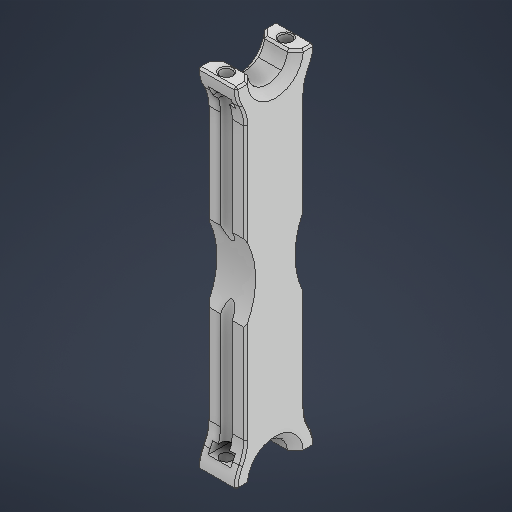
# Autodesk Inventor part: gaffel
Saved by Autodesk Inventor 2026.3 (Build 303398000, 398)
## iProperties
Created: 2026-05-02
Part Number: gaffel
Material: Generic
Document SubType Name: Modeling
Designer: frede
Density: 1 g/cm^3
Appearance: Default
Author: frede
Autodesk Inventor part; units mm, degrees
ref_plane "YZ Plane" through (0, 0, 0) normal (1, 0, 0) x (0, 1, 0)
sketch "Sketch1" plane through (0, 0, 0) normal (1, 0, 0) x (0, 1, 0)
  circle A0 centre (0, 0) radius 5.1
  circle A1 centre (88.4, 0) radius 5.1
  arc A2 (6.6144, 7.5) -> (6.6144, -7.5) centre (0, 0) ccw
  arc A3 (81.7856, -7.5) -> (81.7856, 7.5) centre (88.4, 0) ccw
  line L0 (10, 0) -> (78.4, 0)
  line L1 (81.7856, -7.5) -> (6.6144, -7.5)
  line L2 (6.6144, 7.5) -> (81.7856, 7.5)
  line L3 (81.7, -7.5) -> (6.7, 7.5) construction
  line L4 (6.7, -7.5) -> (81.7, 7.5) construction
  line L5 (0, 10) -> (0, 5.1)
  line L6 (0, -5.1) -> (0, -10)
  line L7 (88.4, -10) -> (88.4, -5.1)
  line L8 (88.4, 5.1) -> (88.4, 10)
  point P0 (44.2, 0)
  dimension "d0" = 10.2
  dimension "d1" = 10.2
  dimension "d2" = 20
  dimension "d3" = 20
  dimension "d6" = 15
  dimension "d42" = 88.4
  constraints: 18 end point, 12 point on circle, 8 point on line, 4 centre point, 3 coincident, 3 midpoint, 2 horizontal, 1 parallel, 1 vertical, 1 other
  measures "d0" diameter of A0
  measures "d1" diameter of A1
  measures "d2" diameter of A2
  measures "d3" diameter of A3
  measures "d6" distance between parallel lines of L1 L2
  measures "d42" distance of point (0, 0) A1.centre
extrude "Extrusion1" add sketch "Sketch1" along normal blind 9.8 contours A0 L5 A2 L2 A3 L8 A1 L7 L1 L6
fillet "Fillet1" radius 10 4 edges at (4.9, 81.7856, 7.5) (4.9, 81.7856, -7.5) (4.9, 6.6144, -7.5) (4.9, 6.6144, 7.5)
chamfer "Chamfer4" distance 2 angle 45 4 edges at (9.8, 83.3, 0) (0, 83.3, 0) (9.8, 5.1, 0) (0, 5.1, 0)
chamfer "Chamfer5" distance 0.5 angle 45 36 edges at (9.8, 44.2, 7.5) (9.8, 2.5, 9.6825) (9.8, 85.9, 9.6825) (0, 2.5, 9.6825) (0, 44.2, 7.5) (0, 85.9, 9.6825) (9.8, 44.2, -7.5) (9.8, 85.9, -9.6825) (9.8, 2.5, -9.6825) (0, 44.2, -7.5) (0, 85.9, -9.6825) (0, 2.5, -9.6825) (9.8, 0, -8.55) (8.8, 0, -6.1) (4.9, 0, -5.1) (1, 0, -6.1) (0, 0, -8.55) (4.9, 0, -10) (4.9, 0, 5.1) (8.8, 0, 6.1) (9.8, 0, 8.55) (4.9, 0, 10) (0, 0, 8.55) (1, 0, 6.1) (8.8, 88.4, 6.1) (9.8, 88.4, 8.55) (4.9, 88.4, 10) (0, 88.4, 8.55) (1, 88.4, 6.1) (4.9, 88.4, 5.1) (4.9, 88.4, -5.1) (8.8, 88.4, -6.1) (9.8, 88.4, -8.55) (4.9, 88.4, -10) (0, 88.4, -8.55) (1, 88.4, -6.1)
sketch "Sketch2" plane through (0.5, 0, 9.5) normal (0, -1, 0) x (1, 0, 0)
  line L0 (8.8, 0) -> (0, 0) projected
  line L1 (4.4, 0) -> (4.4, -3.9)
  line L2 (1.7071, -3.9) -> (7.0929, -3.9) projected
  line L3 (7.0929, -15.1) -> (1.7071, -15.1) projected
  line L4 (4.4, -15.1) -> (4.4, -19)
  line L5 (0, -19) -> (8.8, -19) projected
  point P0 (-0.5, -9.5)
  point P1 (4.4, -17.05)
  point P2 (4.4, -1.95)
  constraints: 4 end point, 4 midpoint
hole "Hole1" at (4.9, 0, -7.55) at (4.9, 0, 7.55) direction (0, 1, 0) diameter 3 end through all countersink diameter 3.5 countersink angle 90
chamfer "Chamfer3" distance 0.25 angle 45 2 edges at (4.9, 88.4, 9.05) (4.9, 88.4, -6.05)
ref_plane "Work Plane1" through (0, 88.4, -10) normal (0, 0, -1) x (-1, 0, 0)
sketch "Sketch3" plane through (0, 88.4, -10) normal (0, 0, -1) x (-1, 0, 0)
  line L0 (-7.775, -3.75) -> (-2.025, -3.75)
  line L1 (-2.025, -3.75) -> (-2.025, -6.25)
  line L2 (-2.025, -6.25) -> (-7.775, -6.25)
  line L3 (-7.775, -6.25) -> (-7.775, -3.75)
  line L4 (-7.775, -3.75) -> (-2.025, -6.25) construction
  line L5 (-2.025, -3.75) -> (-7.775, -6.25) construction
  line L6 (-0.5, 0) -> (-9.3, 0) projected
  line L7 (-9.8, -4.5992) -> (-9.8, -0.5) projected
  point P0 (0, -88.4)
  point P1 (-4.9, -5)
  point P2 (0, -0.5)
  dimension "d27" = 5.75
  dimension "d28" = 2.5
  dimension "d39" = 5
  dimension "d40" = 4.9
  dimension "d41" = 9.8
  constraints: 12 end point, 2 midpoint, 2 parallel, 1 horizontal, 1 perpendicular
  measures "d27" distance of L1.end L2.end
  measures "d28" distance of L0.end L1.end
  measures "d39" distance from line of L6 point (-4.9, -5)
  measures "d40" distance from line of L7 point (-4.9, -5)
  measures "d41" distance of point (0, -0.5) L7.end
extrude "Extrusion2" cut sketch "Sketch3" against normal blind 6.5
ref_plane "Work Plane2" through (3.4008, 44.2, -7.5) normal (0, 1, 0) x (1, 0, 0)
mirror "Mirror1" about plane through (0, 0, 0) normal (0, 0, 1) of "Extrusion2"
mirror "Mirror2" about plane through (3.4008, 44.2, -7.5) normal (0, 1, 0) of "Extrusion2", "Mirror1"
sketch "Sketch4" plane through (9.8, 0, 0) normal (1, 0, 0) x (0, 0, -1)
  arc A0 (-5.0755, 87.9003) -> (5.0755, 87.9003) centre (0, 88.4) ccw projected
  line L0 (0, 88.4) -> (0, 0)
  circle A1 centre (0, 44.2) radius 25
  circle A2 centre (-25, 44.2) radius 20
  circle A3 centre (25, 44.2) radius 20
  point P0 (17, 62.5303)
  point P1 (17, 25.8697)
  point P2 (-17, 62.5303)
  point P3 (-17, 25.8697)
  dimension "d43" = 50
  dimension "d44" = 40
  dimension "d45" = 40
  constraints: 3 centre point, 2 end point, 2 point on circle, 1 midpoint, 1 vertical
  measures "d43" diameter of A1
  measures "d44" diameter of A2
  measures "d45" diameter of A3
extrude "Extrusion3" cut sketch "Sketch4" against normal up to surface (9.8 mm away) contours A1 A3 | A2 A1 picked at (18.3359, 40.9655) picked at (-18.2183, 44.2)
equation "\"d40\" = 0.5 * d41"
equation "\"d45\" = d44"
body "Solid1"
